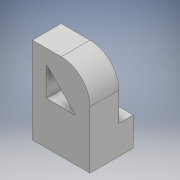
# Autodesk Inventor part: 37
Saved by Autodesk Inventor 2017 (Build 210142000, 142)
## iProperties
Part Number: 37
Material: 一般
Document SubType Name: Modeling
Designer: Brian
Density: 1 g/cm^3
Appearance: 預設
Author: Brian
Autodesk Inventor part; units mm, degrees
ref_plane "YZ Plane" through (0, 0, 0) normal (1, 0, 0) x (0, 1, 0)
ref_plane "XZ Plane" through (0, 0, 0) normal (0, 1, 0) x (-1, 0, 0)
ref_plane "XY Plane" through (0, 0, 0) normal (0, 0, 1) x (1, 0, 0)
sketch "草圖1" plane through (0, 0, 0) normal (0, 1, 0) x (-1, 0, 0)
  line L0 (0, 0) -> (-40, 0)
  line L1 (-40, 0) -> (-40, -60)
  line L2 (-40, -60) -> (0, -60)
  line L3 (0, -60) -> (0, 0)
  line L4 (-10, -30) -> (-30, -30)
  line L5 (-30, -30) -> (-30, -10)
  line L6 (-30, -10) -> (-10, -10)
  line L7 (-10, -10) -> (-10, -30)
  dimension "d0" = 10
  dimension "d1" = 10
  dimension "d2" = 20
  dimension "d3" = 60
  dimension "d4" = 20
  dimension "d5" = 10
  constraints: 16 end point, 4 parallel, 2 horizontal, 2 perpendicular
  measures "d0" distance between parallel lines of L3 L7
  measures "d1" distance between parallel lines of L1 L5
  measures "d2" distance of L4.start L4.end
  measures "d3" distance of L0.end L1.end
  measures "d4" distance of L4.end L5.end
  measures "d5" distance between parallel lines of L0 L6
extrude "擠出1" add sketch "草圖1" along normal blind 20
sketch "草圖2" plane through (40, 0, -60) normal (0, 0, -1) x (-1, 0, 0)
  line L0 (0, 20) -> (40, 20) projected
  line L1 (40, 20) -> (0, 20) projected
  line L2 (0, 20) -> (0, 30)
  line L3 (0, 30) -> (10, 30)
  line L4 (10, 30) -> (30, 40)
  line L5 (30, 40) -> (40, 40)
  line L6 (40, 40) -> (40, 20)
  point P0 (40, 0)
  dimension "d8" = 10
  dimension "d9" = 10
  dimension "d10" = 20
  dimension "d11" = 20
  constraints: 10 end point, 2 perpendicular, 1 horizontal, 1 vertical
  measures "d8" distance of L0.start L2.end
  measures "d9" distance of L2.end L3.end
  measures "d10" horizontal distance of L3.end L4.end
  measures "d11" distance of L5.end L0.end
extrude "擠出2" add sketch "草圖2" against normal blind 20
chamfer "倒角1" distance 20 angle 45 1 edges at (30, 10, -10)
fillet "圓角1" radius 20 1 edges at (40, 10, 0)
